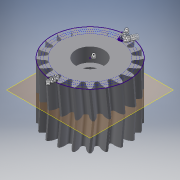
# Autodesk Inventor part: gear 4 idler herring
Saved by Autodesk Inventor 2017 (Build 210142000, 142)
## iProperties
Created: 2018-04-17
Part Number: gear 4 idler herring
Material: Generic
Document SubType Name: Modeling
Designer: RKL
Density: 1 g/cm^3
Appearance: Default
Author: RKL
Autodesk Inventor part; units mm, degrees
ref_plane "YZ Plane" through (0, 0, 0) normal (1, 0, 0) x (0, 1, 0)
ref_plane "XZ Plane" through (0, 0, 0) normal (0, 1, 0) x (-1, 0, 0)
ref_plane "XY Plane" through (0, 0, 0) normal (0, 0, 1) x (1, 0, 0)
sketch "Sketch1" plane through (0, 0, 0) normal (0, 0, 1) x (1, 0, 0)
  spline S0 degree 3 poles (-1.8364, 13.6259) (-1.7252, 13.4828) (-1.503, 13.1968) (-1.2179, 12.7331) (-1.0222, 12.3244) (-0.8976, 11.9835) (-0.8637, 11.8055) (-0.8468, 11.7165) knots 0 0 0 0 0.250051 0.500092 0.750067 0.875095 1 1 1 1
  spline S1 degree 3 poles (-0.8468, 11.7165) (-0.8422, 11.6524) (-0.8329, 11.5241) (-0.7964, 11.3345) (-0.7411, 11.1494) (-0.6555, 10.9757) (-0.5352, 10.823) (-0.3784, 10.7082) (-0.1935, 10.6415) (0, 10.647) (0.1935, 10.6415) (0.3784, 10.7082) (0.5352, 10.823) (0.6555, 10.9757) (0.7411, 11.1494) (0.7964, 11.3345) (0.8329, 11.5241) (0.8422, 11.6524) (0.8468, 11.7165) knots 0 0 0 0 0.062584 0.125166 0.187726 0.250287 0.31277 0.375174 0.437496 0.5 0.562504 0.624826 0.68723 0.749713 0.812274 0.874834 0.937416 1 1 1 1
  spline S2 degree 3 poles (0.8468, 11.7165) (0.8637, 11.8055) (0.8976, 11.9835) (1.0222, 12.3244) (1.2179, 12.7331) (1.503, 13.1968) (1.7252, 13.4828) (1.8364, 13.6259) knots 0 0 0 0 0.124905 0.249933 0.499908 0.749949 1 1 1 1
  circle A0 centre (0, 0) radius 10.6451 construction
  circle A1 centre (0, 0) radius 11.7462 construction
  circle A2 centre (0, 0) radius 12.5 construction
  circle A3 centre (0, 0) radius 13.7491
  point P0 (-1.511, 13.191)
  point P1 (-1.2262, 12.7286)
  point P2 (-0.9937, 12.2381)
  point P3 (-0.9047, 11.9815)
  point P4 (-0.8291, 11.5246)
  point P5 (-0.7932, 11.3352)
  point P6 (-0.7361, 11.1513)
  point P7 (-0.6497, 10.9791)
  point P8 (-0.529, 10.8292)
  point P9 (-0.3737, 10.7162)
  point P10 (-0.1923, 10.6535)
  point P11 (0, 10.6451)
  point P12 (0.1923, 10.6535)
  point P13 (0.3737, 10.7162)
  point P14 (0.529, 10.8292)
  point P15 (0.6497, 10.9791)
  point P16 (0.7361, 11.1513)
  point P17 (0.7932, 11.3352)
  point P18 (0.8291, 11.5246)
  point P19 (0.9047, 11.9815)
  point P20 (0.9937, 12.2381)
  point P21 (1.2262, 12.7286)
  point P22 (1.511, 13.191)
  constraints: 4 centre point, 2 point on circle, 61 other
extrude "Extrusion1" add sketch "Sketch1" against normal blind 20
extrude "Extrusion2" [suppressed]
pattern_circular "Circular Pattern1" [suppressed]
sketch "Sketch2" plane through (0, 0, 0) normal (0, 0, 1) x (1, 0, 0)
  circle A0 centre (0, 0) radius 5
  dimension "d7" = 10
  constraints: 1 centre point, 1 coincident
  measures "d7" diameter of A0
extrude "Extrusion3" cut sketch "Sketch2" against normal blind 5
sketch "Sketch3" plane through (0, 0, -5) normal (0, 0, 1) x (1, 0, 0)
  circle A0 centre (0, 0) radius 3
  dimension "d10" = 6
  constraints: 1 centre point, 1 coincident
  measures "d10" diameter of A0
extrude "Extrusion4" cut sketch "Sketch3" against normal through all
ref_plane "Work Plane1" through (0, 0, -10) normal (0, 0, 1) x (1, 0, 0)
mirror "Mirror1" about plane through (0, 0, -10) normal (0, 0, 1) of "Extrusion3"
coil "Coil1" sketch "Sketch1" operation cut axis through (0, 0, -10) along (0, 0, -1) pitch 1000 turns 0.01 hand left contours A3 S2 S1 S0
sketch "Sketch4" plane through (0, 0, -10) normal (0, 0, 1) x (0.9980267, 0.0627905, 0)
  circle A0 centre (0, 0) radius 12.5 construction
  spline S0 degree 3 poles (-0.8468, 11.7165) (-0.8637, 11.8055) (-0.8976, 11.9835) (-1.0222, 12.3244) (-1.2179, 12.7331) (-1.503, 13.1968) (-1.7252, 13.4828) (-1.8364, 13.6259) knots 0 0 0 0 0.124905 0.249933 0.499908 0.749949 1 1 1 1 projected
  spline S1 degree 3 poles (0.8468, 11.7165) (0.8422, 11.6524) (0.8329, 11.5241) (0.7964, 11.3345) (0.7411, 11.1494) (0.6555, 10.9757) (0.5352, 10.823) (0.3784, 10.7082) (0.1935, 10.6415) (0, 10.647) (-0.1935, 10.6415) (-0.3784, 10.7082) (-0.5352, 10.823) (-0.6555, 10.9757) (-0.7411, 11.1494) (-0.7964, 11.3345) (-0.8329, 11.5241) (-0.8422, 11.6524) (-0.8468, 11.7165) knots 0 0 0 0 0.062584 0.125166 0.187726 0.250287 0.31277 0.375174 0.437496 0.5 0.562504 0.624826 0.68723 0.749713 0.812274 0.874834 0.937416 1 1 1 1 projected
  spline S2 degree 3 poles (1.8364, 13.6259) (1.7252, 13.4828) (1.503, 13.1968) (1.2179, 12.7331) (1.0222, 12.3244) (0.8976, 11.9835) (0.8637, 11.8055) (0.8468, 11.7165) knots 0 0 0 0 0.250051 0.500092 0.750067 0.875095 1 1 1 1 projected
  arc A1 (1.8364, 13.6259) -> (-1.8364, 13.6259) centre (0, 0) ccw projected
  constraints: 1 horizontal alignment, 2 other
coil "Coil2" sketch "Sketch4" operation cut axis through (0, 0, -10) along (0, 0, -1) pitch 1000 turns 0.01 hand right
pattern_circular "Circular Pattern2" count 20 over 360 about axis through (0, 0, 0) along (0, 0, -1) of "Coil1", "Coil2"
equation "\"d0\" = FaceWidth"
equation "\"Module\" = 1.25"
equation "\"PressureAngle\" = 20deg"
equation "\"UnitProfileClearance\" = 0.25"
equation "\"UnitRoundRadius\" = 0.35"
equation "\"HeadDiameter\" = 27.49812"
equation "\"RootDiameter\" = 21.29024"
equation "\"BaseDiameter\" = 23.49232"
equation "\"PitchDiameter\" = 25"
equation "\"FaceWidth\" = 20"
equation "\"HelixAngle\" = 0"
equation "\"UnitCorrection\" = 0"
equation "\"UnitAddendumModification\" = 0.000753"
equation "\"CircularPitch\" = 3.926991"
equation "\"UnitBacklashShift\" = -0.233904"
equation "\"TotalToolShift\" = -0.29238"
equation "\"IsInternal\" = 0"
body "Solid1"
